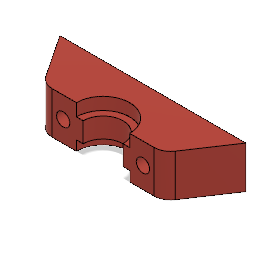
X-carriage-III-part3-rev2 v4 (Autodesk Fusion 360 design; units mm, degrees)
Autodesk Fusion 360 part; units mm, degrees
note: some values were not read from the file. Set by a fixed rule: which sketch regions a step uses.
sketch "Sketch1" plane through (0, 0, 0) normal (0, 1, 0) x (1, 0, 0)
  line L0 (-18, 0) -> (-28, 15)
  line L1 (-28, 15) -> (28, 15)
  line L2 (28, 15) -> (18, 0)
  line L3 (18, 0) -> (-18, 0)
  dimension "d1" = 10
  dimension "d2" = 10
  dimension "d3" = 56
  dimension "d21" = 15
extrude "Extrude1" add sketch "Sketch1" along normal blind 12.7
sketch "Sketch2" plane through (0, 12.7, 0) normal (0, 1, 0) x (-1, 0, 0)
  line L0 (-18, 0) -> (-28, -15)
  line L1 (-28, -15) -> (28, -15)
  line L2 (28, -15) -> (18, 0)
  line L3 (18, 0) -> (-18, 0)
  circle A0 centre (0, 0) radius 8
  circle A1 centre (0, 0) radius 6
  dimension "d7" = 16
  dimension "d8" = 12
  measures "d7" diameter of A0
  measures "d8" diameter of A1
extrude "Extrude2" cut sketch "Sketch2" against normal through all contours L3 A1 picked at (-1.4661, -1.3603)
extrude "Extrude3" cut sketch "Sketch2" against normal blind 3.7 contours L3 A0 A1 picked at (7.2812, -0.6955)
extrude "Extrude4" cut sketch "Sketch2" along normal blind 3 from surface at -12.7 contours L3 A0 A1 picked at (7.2812, -0.6955)
sketch "Sketch3" plane through (0, 0, 0) normal (0, 0, 1) x (1, 0, 0)
  line L0 (-8, 3) -> (-6, 3)
  line L1 (-6, 3) -> (-6, 9)
  line L2 (-6, 9) -> (-8, 9)
  line L3 (-8, 9) -> (-8, 12.7)
  line L4 (-8, 12.7) -> (-18, 12.7)
  line L5 (-18, 12.7) -> (-18, 0)
  line L6 (-18, 0) -> (-8, 0)
  line L7 (-8, 0) -> (-8, 3)
  line L8 (-12, 6.35) -> (12, 6.35)
  circle A0 centre (-12, 6.35) radius 2
  circle A1 centre (12, 6.35) radius 2
  dimension "d15" = 24
  dimension "d16" = 12
  dimension "d17" = 6.35
  dimension "d18" = 4
  dimension "d19" = 4
  measures "d16" distance of origin
  measures "d17" distance of origin
  measures "d18" diameter of A0
  measures "d19" diameter of A1
extrude "Extrude5" cut sketch "Sketch3" against normal through all contours A0 | A1
fillet "Fillet1" radius 5 2 edges at (-18, 6.35, 0) (18, 6.35, 0)
equation "d17 = ( 12.7 / 2 ) * 1 mm"
